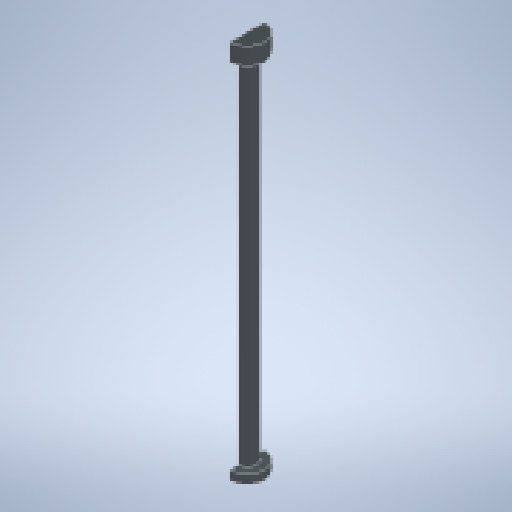
# Autodesk Inventor part: Rod
Saved by Autodesk Inventor 2025.1 (Build 291241000, 241)
## iProperties
Created: 2024-10-22
Part Number: Rod
Material: Generic
Document SubType Name: Modeling
Designer: vedan
Density: 1 g/cm^3
Appearance: Iron Gray
Author: vedan
Autodesk Inventor part; units mm, degrees
ref_plane "YZ Plane" through (0, 0, 0) normal (1, 0, 0) x (0, 1, 0)
ref_plane "XZ Plane" through (0, 0, 0) normal (0, 1, 0) x (-1, 0, 0)
ref_plane "XY Plane" through (0, 0, 0) normal (0, 0, 1) x (1, 0, 0)
sketch "Sketch1" plane through (0, 0, 0) normal (0, 0, 1) x (1, 0, 0)
  line L0 (0, 0) -> (2.5, 0)
  line L1 (2.5, 0) -> (2.5, 107.3)
  line L2 (2.5, 107.3) -> (0, 107.3)
  line L3 (0, 107.3) -> (0, 0)
  line L4 (0, 107.3) -> (5, 107.3)
  line L5 (5, 107.3) -> (5, 104.8)
  line L6 (5, 104.8) -> (0, 104.8)
  line L7 (0, 104.8) -> (0, 107.3)
  line L8 (0, 0) -> (5, 0)
  line L9 (5, 0) -> (5, 2.5)
  line L10 (5, 2.5) -> (0, 2.5)
  line L11 (0, 2.5) -> (0, 0)
  point P0 (2.5, 2.5)
  point P1 (2.5, 104.8)
  dimension "d0" = 2.5
  dimension "d1" = 107.3
  dimension "d2" = 5
  dimension "d3" = 2.5
  dimension "d4" = 5
  dimension "d5" = 2.5
  constraints: 24 end point, 6 parallel, 3 horizontal, 3 perpendicular
  measures "d0" distance of L2.end L1.end
  measures "d1" distance of L1.end L0.end
  measures "d2" distance of L5.end L6.end
  measures "d3" distance of L4.end L5.end
  measures "d4" distance of L10.end L9.end
  measures "d5" distance of L9.end L8.end
revolve "Revolution1" add sketch "Sketch1" angle 360 about axis through (0, 107.3, 0) along (0, -1, 0)
sketch "Sketch4" plane through (0, 107.3, 0) normal (0, 1, 0) x (1, 0, 0)
  circle A0 centre (0, 0) radius 5 projected
  line L0 (0, -5) -> (0, 5)
  arc A1 (0, 5) -> (0, -5) centre (0, 0) ccw
  constraints: 4 point on circle, 2 end point, 1 centre point, 1 coincident, 1 concentric, 1 vertical
extrude "Extrusion3" cut sketch "Sketch4" against normal through all contours L0 A0 picked at (-0.7745, -1.4758)
sketch "Sketch5" plane through (0, 107.3, 0) normal (0, 1, 0) x (1, 0, 0)
  arc A0 (0, -5) -> (0, 5) centre (0, 0) ccw
  line L0 (0, -5) -> (0, 5)
  constraints: 2 end point, 2 point on circle, 1 centre point, 1 coincident, 1 vertical
extrude "Extrusion4" add sketch "Sketch5" along normal blind 4
body "Solid1"
